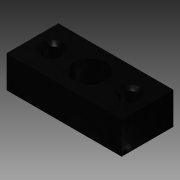
# Autodesk Inventor part: supporto guide x
Saved by Autodesk Inventor 2014 SP1 (Build 180222100, 222)
## iProperties
Created: 2015-04-08
Part Number: supporto guide x
Material: Generic
Document SubType Name: Modeling
Designer: Giorgio Nuzzo
Density: 1 g/cm^3
Appearance: Fine Textured - Black
d0: 16,200 mm
d1: 36,000 mm
d2: 10,000 mm
d3: 5,100 mm
d4: 12,000 mm
d5: 5,100 mm
d6: 12,000 mm
d7: 10,000 mm
d8: 0,00 deg
d9: 1,000 mm
Author: Giorgio Nuzzo
Autodesk Inventor part; units mm, degrees
ref_plane "YZ Plane" through (0, 0, 0) normal (1, 0, 0) x (0, 1, 0)
ref_plane "XZ Plane" through (0, 0, 0) normal (0, 1, 0) x (-1, 0, 0)
ref_plane "XY Plane" through (0, 0, 0) normal (0, 0, 1) x (1, 0, 0)
sketch "Sketch1" plane through (0, 0, 0) normal (0, 0, 1) x (1, 0, 0)
  line L0 (-18, 8.1) -> (18, 8.1)
  line L1 (18, 8.1) -> (18, -8.1)
  line L2 (18, -8.1) -> (-18, -8.1)
  line L3 (-18, -8.1) -> (-18, 8.1)
  line L4 (0, 11.34) -> (0, -11.34) construction
  line L5 (-25.2, 0) -> (25.2, 0) construction
  circle A0 centre (0, 0) radius 5
  circle A1 centre (-12, 0) radius 2.55
  circle A2 centre (12, 0) radius 2.55
  dimension "d0" = 16.2
  dimension "d1" = 36
  dimension "d2" = 10
  dimension "d3" = 5.1
  dimension "d4" = 12
  dimension "d5" = 5.1
  dimension "d6" = 12
  constraints: 8 end point, 3 centre point, 2 parallel, 2 point on line, 1 coincident, 1 horizontal, 1 perpendicular, 2 other
  measures "d0" distance of L2.end L0.start
  measures "d1" distance of L0.start L0.end
  measures "d2" diameter of A0
  measures "d3" diameter of A1
  measures "d4" distance of A0.centre A1.centre
  measures "d5" diameter of A2
  measures "d6" distance of A0.centre A2.centre
extrude "Extrusion1" add sketch "Sketch1" along normal blind 10
chamfer "Chamfer1" distance 1 angle 45 2 edges at (-14.55, 0, 10) (9.45, 0, 10)
equation "\"d5\" = d3"
equation "\"d6\" = d4"
body "Solid1"
